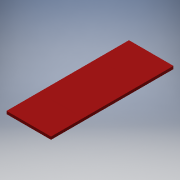
# Autodesk Inventor part: bottom rail cover
Saved by Autodesk Inventor 2018.1 (Build 221171000, 171)
## iProperties
Created: 2017-11-13
Part Number: bottom rail cover
Material: ABS-Kunststoff
Document SubType Name: Modeling
Designer: tillm
Density: 1.06 g/cm^3
Appearance: Rot
Author: tillm
Autodesk Inventor part; units mm, degrees
ref_plane "YZ Plane" through (0, 0, 0) normal (1, 0, 0) x (0, 1, 0)
ref_plane "XZ Plane" through (0, 0, 0) normal (0, 1, 0) x (-1, 0, 0)
ref_plane "XY Plane" through (0, 0, 0) normal (0, 0, 1) x (1, 0, 0)
sketch "Skizze1" plane through (0, 0, 0) normal (0, 0, 1) x (1, 0, 0)
  line L0 (40, 110) -> (-40, 110)
  line L1 (-40, 110) -> (-40, -110)
  line L2 (-40, -110) -> (40, -110)
  line L3 (40, -110) -> (40, 110)
  line L4 (40, 110) -> (-40, -110) construction
  line L5 (-40, 110) -> (40, -110) construction
  point P0 (0, 0)
  dimension "d0" = 80
  dimension "d1" = 220
  constraints: 12 end point, 2 midpoint, 2 parallel, 1 horizontal, 1 perpendicular
  measures "d0" distance of L2.end L1.end
  measures "d1" distance of L1.end L0.end
extrude "Extrusion1" add sketch "Skizze1" along normal blind 5
sketch "Skizze2" plane through (0, 0, 5) normal (0, 0, 1) x (1, 0, 0)
  circle A0 centre (-2.5, -74) radius 4 projected
  circle A1 centre (-2.5, 76) radius 4 projected
  line L0 (-40, 110) -> (-40, -110) projected
  line L1 (-40, -86) -> (5, -86)
  line L2 (-40, -61) -> (5, -61)
  line L3 (-40, -110) -> (40, -110) projected
  arc A2 (5, -86) -> (5, -61) centre (5, -73.5) ccw
  line L4 (-40, -35) -> (-15, -35)
  line L5 (-15, -35) -> (-15, 35)
  line L6 (-15, 35) -> (-40, 35)
  line L7 (-40, 35) -> (-40, -35)
  line L8 (-74.8767, 0) -> (54.4442, 0)
  line L9 (-40, 86) -> (5, 86)
  line L10 (-40, 61) -> (5, 61)
  arc A3 (5, 61) -> (5, 86) centre (5, 73.5) ccw
  line L11 (-15, -10) -> (10, -10)
  line L12 (-15, 10) -> (10, 10)
  arc A4 (10, -10) -> (10, 10) centre (10, 0) ccw
  line L13 (-40, 61) -> (-40, 86)
  point P0 (0, 0)
  dimension "d4" = 45
  dimension "d5" = 45
  dimension "d6" = 24
  dimension "d7" = 25
  dimension "d8" = 0
  dimension "d9" = 25
  dimension "d10" = 70
  dimension "d11" = 75
  dimension "d12" = 25
  dimension "d13" = 25
  dimension "d14" = 20
  dimension "d15" = 25
  constraints: 24 end point, 6 point on circle, 6 point on line, 5 horizontal, 5 symmetric about line, 3 centre point, 3 parallel, 1 perpendicular, 1 vertical, 1 other
  measures "d4" distance of L1.start L1.end
  measures "d5" distance of L2.start L2.end
  measures "d6" distance between parallel lines of L3 L1
  measures "d7" distance between parallel lines of L2 L1
  measures "d8" horizontal distance of L1.end A2.centre
  measures "d9" distance of L6.end L5.end
  measures "d10" distance of L5.end L4.end
  measures "d11" distance between parallel lines of L3 L4
  measures "d12" distance of L11.start L11.end
  measures "d13" distance of L12.start L12.end
  measures "d14" distance between parallel lines of L12 L11
  measures "d15" distance from line of L5.end L12
extrude "Extrusion2" cut sketch "Skizze2" against normal up to next contours A0 | A1 | L9 A3 L10 L0 | L2 A2 L1 L0 | L6 L5 L8 L0 | L8 L5 L4 L0 | L8 A4 L11 L5 | L5 L12 A4 L8
